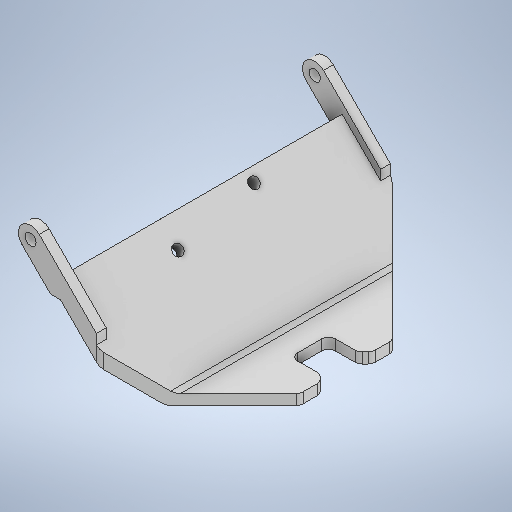
# Autodesk Inventor part: FrontLock
Saved by Autodesk Inventor 2025.1 (Build 291241000, 241)
## iProperties
Created: 2026-05-10
Part Number: FrontLock
Material: Generic
Document SubType Name: Modeling
Designer: User
Density: 1 g/cm^3
Appearance: Default
Author: User
## iProperties of the stored document FrontLock_3DPrint.ipt
Created: 2026-05-12
Part Number: FrontLock_3DPrint
Material: Generic
Document SubType Name: Modeling
Designer: User
Density: 1 g/cm^3
Appearance: Default
Author: User
Autodesk Inventor part; units mm, degrees
ref_plane "YZ Plane" through (0, 0, 0) normal (1, 0, 0) x (0, 1, 0)
sketch "Sketch1" plane through (0, 0, 0) normal (0, 0, 1) x (1, 0, 0)
  circle A0 centre (-6.485281, 1.485281) radius 1.5
  circle A1 centre (-6.485281, 1.485281) radius 1.6
  line L0 (4, 5) -> (-10, 5)
  line L1 (-10, 5) -> (-10, -7)
  line L2 (-3, 0) -> (-5, -2)
  circle A2 centre (-6.485281, 1.485281) radius 3.514719
  line L3 (54.104764, -60.437628) -> (54.104764, 0)
  line L4 (-6.485281, 1.485281) -> (54.104764, -59.104764)
  line L5 (-6.485281, 1.485281) -> (79.201983, 1.485281) construction
  line L6 (-10, -7) -> (-5, -7)
  line L7 (-5, -2) -> (-3, 0)
  line L8 (-5, -2) -> (-3, 0)
  line L9 (-5, -7.5) -> (-10.5, -7.5)
  line L10 (-10.5, -7.5) -> (-10.5, 5.5)
  line L11 (-10.5, 5.5) -> (4, 5.5)
  line L12 (-2.646447, -0.353553) -> (-4.646447, -2.353553)
  circle A3 centre (-6.485281, 1.485281) radius 9.107214
  circle A4 centre (-6.485281, 1.485281) radius 9.841405
  line L13 (0.473643, -5.473643) -> (-0.587018, -6.534303)
  line L14 (0.473643, -5.473643) -> (1.973643, -5.473643) construction
  line L15 (-0.587018, -6.534303) -> (1.534303, -4.412982)
  line L16 (23.809741, -28.809741) -> (24.870402, -27.749081)
  line L17 (1.534303, -4.412982) -> (-0.587018, -6.534303)
  line L18 (-0.587018, -6.534303) -> (22.749081, -29.870402)
  line L19 (22.749081, -29.870402) -> (24.870402, -27.749081)
  line L20 (24.870402, -27.749081) -> (1.534303, -4.412982)
  line L21 (-0.587018, -6.534303) -> (1.534303, -4.412982)
  line L22 (1.534303, -4.412982) -> (-3.826704, 0.948024)
  line L23 (-3.826704, 0.948024) -> (-5.948024, -1.173296)
  line L24 (-5.948024, -1.173296) -> (-0.587018, -6.534303)
  line L25 (22.749081, -29.870402) -> (54.104764, -29.870402)
  line L26 (54.104764, -29.870402) -> (54.104764, -26.870402)
  line L27 (54.104764, -26.870402) -> (22.749081, -26.870402)
  line L28 (22.749081, -26.870402) -> (22.749081, -29.870402)
  point P0 (0, 0)
  point P1 (-3.17704, 0.29836)
  point P2 (-5.29836, -1.822961)
  point P3 (23.991722, -26.870402)
extrude "Extrusion1" add sketch "Sketch1" along normal blind 3 contours A2 L22 L23 L24 | L22 L15 A4 | A4 L4 A3 L22 | A3 L4 A2 L22 | A4 L24 A3 L4 | L15 L20 L27 L28 L4 | L13 L24 A4 | L4 L28 L18 L13 | A2 L4 L23 L22 | L24 L23 L4 A2 | A2 L4 A3 L24 | L28 L27 L20 L16 L4 | L4 L19 L28 | L27 L3 L25 L4 L16 L20 | L4 L25 L19
sketch "Sketch2" plane through (0, 0, 0) normal (0, 0, -1) x (-1, 0, 0)
  line L0 (10, -7) -> (5, -7)
  line L1 (5.29836, -1.822961) -> (-22.749081, -29.870402)
  arc A0 (5.29836, -1.822961) -> (3.17704, 0.29836) centre (6.485281, 1.485281) ccw
  line L2 (-23.991722, -26.870402) -> (3.17704, 0.29836)
  line L3 (-54.104764, -26.870402) -> (-23.991722, -26.870402)
  line L4 (-54.104764, -29.870402) -> (-54.104764, -26.870402)
  line L5 (-22.749081, -29.870402) -> (-54.104764, -29.870402)
  circle A1 centre (6.485281, 1.485281) radius 1.6
  circle A2 centre (6.485281, 1.485281) radius 9.184402
  circle A3 centre (6.485281, 1.485281) radius 9.684402
  point P0 (0, 0)
  point P1 (-1.340645, -4.219325)
  point P2 (0.780675, -6.340645)
  dimension "d11" = 0.5
  constraints: 1 centre point, 1 coincident, 3 other
extrude "Extrusion2" cut sketch "Sketch2" against normal blind 0.2 contours L1 A2 L2 A0 | L1 A3 L2 A2 picked at (2.707023, -2.056333) picked at (0.758356, -5.892503)
sketch "Sketch3" plane through (0, 0, 0) normal (0, 0, -1) x (-1, 0, 0)
  arc A0 (-1.340645, -4.219325) -> (0.780675, -6.340645) centre (6.485281, 1.485281) ccw
  line L0 (-23.991722, -26.870402) -> (-1.340645, -4.219325)
  line L1 (-54.104764, -26.870402) -> (-23.991722, -26.870402)
  line L2 (-54.104764, -29.870402) -> (-54.104764, -26.870402)
  line L3 (-22.749081, -29.870402) -> (-54.104764, -29.870402)
  line L4 (0.780675, -6.340645) -> (-22.749081, -29.870402)
  point P0 (0, 0)
ref_plane "Work Plane1" through (-10, -7, -78.180224) normal (0, 0, -1) x (0, 1, 0)
extrude "Extrusion3" add sketch "Sketch3" along normal up to surface (78.180224 mm away)
sketch "Sketch4" plane through (54.104764, -29.870402, -78.180224) normal (0, 0, -1) x (-1, 0, 0)
  line L0 (30.113042, 3) -> (52.764119, 25.651077)
  line L1 (0, 3) -> (30.113042, 3)
  line L2 (0, 0) -> (0, 3)
  line L3 (31.355683, 0) -> (0, 0)
  line L4 (54.88544, 23.529757) -> (31.355683, 0)
  arc A0 (52.764119, 25.651077) -> (54.88544, 23.529757) centre (60.590046, 31.355683) ccw
  point P0 (54.104764, 29.870402)
extrude "Extrusion4" add sketch "Sketch4" along normal blind 0.2
sketch "Sketch6" plane through (54.104764, -29.870402, -78.380224) normal (0, 0, -1) x (-1, 0, 0)
  line L0 (59.403124, 28.047441) -> (31.355683, 0)
  line L1 (31.355683, 0) -> (0, 0)
  line L2 (0, 0) -> (0, 3)
  line L3 (0, 3) -> (30.113042, 3)
  line L4 (30.113042, 3) -> (57.281804, 30.168762)
  arc A0 (59.403124, 28.047441) -> (57.281804, 30.168762) centre (60.590046, 31.355683) ccw
  circle A1 centre (60.590046, 31.355683) radius 1.6
  point P0 (54.104764, 29.870402)
extrude "Extrusion5" add sketch "Sketch6" along normal blind 2.8
sketch "Sketch7" plane through (22.749081, -29.870402, 3) normal (0, -1, 0) x (1, 0, 0)
  line L0 (9.199091, -15.919764) -> (19.199091, -25.919764)
  line L1 (-21.577508, 14.856835) -> (9.199091, -15.919764)
  line L2 (19.199091, -57.937302) -> (9.199091, -67.937302)
  line L3 (-21.577508, -98.713901) -> (9.199091, -67.937302)
  line L4 (0, -84.180224) -> (-28.047441, -84.180224)
  line L5 (31.355683, -84.180224) -> (0, -84.180224)
  line L6 (31.355683, -84.180224) -> (31.355683, 0)
  line L7 (0, 0) -> (31.355683, 0)
  line L8 (-28.047441, 0) -> (0, 0)
  line L9 (19.199091, -25.919764) -> (29.768225, -36.488898)
  line L10 (19.199091, -57.937302) -> (29.743916, -47.392477)
  line L11 (19.199091, -25.919764) -> (19.199091, -57.937302)
  line L12 (19.199091, -25.919764) -> (51.216629, -25.919764) construction
  line L13 (29.768225, -36.488898) -> (29.743916, -47.392477)
  line L14 (29.743916, -47.392477) -> (8.743968, -47.345658)
  line L15 (8.743968, -47.345658) -> (8.768277, -36.442079)
  line L16 (8.768277, -36.442079) -> (29.768225, -36.488898)
  line L17 (-22.991722, 13.442621) -> (7.784877, -17.333978)
  line L18 (7.784877, -17.333978) -> (17.784877, -27.333978)
  line L19 (17.784877, -27.333978) -> (28.354011, -37.903112)
  line L20 (-22.991722, -97.299688) -> (7.784877, -66.523088)
  line L21 (7.784877, -66.523088) -> (17.784877, -56.523088)
  line L22 (17.784877, -56.523088) -> (28.329702, -45.978263)
  point P0 (-22.749081, -3)
  point P1 (-9.549101, 0)
  point P2 (19.199091, -28.748191)
  point P3 (19.199091, -36.465335)
  point P4 (19.199091, -47.368967)
  point P5 (19.199091, -55.108875)
  point P6 (-9.872259, -84.180224)
  dimension "d20" = 90
  dimension "d21" = 21
  dimension "d22" = 2
  dimension "d23" = 2
  constraints: 24 end point, 2 parallel, 2 perpendicular, 1 horizontal, 1 point on line, 4 other
  measures "d20" angle of L11 L12
  measures "d21" distance of L10.end L14.end
  measures "d22" distance between parallel lines of L1 L17
  measures "d23" distance between parallel lines of L3 L20
extrude "Extrusion6" cut sketch "Sketch7" against normal blind 21
chamfer "Chamfer1" distance 2 angle 45 2 edges at (41.9482, -28.3704, -33.4653) (41.9482, -28.3704, -44.369)
fillet "Fillet1" radius 2 12 edges at (31.5174, -28.3704, -33.4421) (39.9482, -28.3704, -33.4609) (41.9482, -28.3704, -31.4653) (31.493, -28.3704, -44.3457) (39.9482, -28.3704, -44.3645) (41.9482, -28.3704, -46.369) (41.9482, -28.3704, -52.1089) (41.9482, -28.3704, -25.7482) (13.2, -18.2, 3) (12.8768, -17.8768, -81.1802) (22.7491, -29.8704, -38.9285) (23.9917, -26.8704, -38.9285)
sketch "Sketch8" plane through (0, 0, 3) normal (0, 0, 1) x (1, 0, 0)
  arc A0 (-3.17704, 0.29836) -> (-5.29836, -1.822961) centre (-6.485281, 1.485281) ccw
  line L0 (-5.29836, -1.822961) -> (12.371554, -19.492874)
  arc A1 (-0.780675, -6.340645) -> (1.340645, -4.219325) centre (-6.485281, 1.485281) ccw
  line L1 (3.678701, -13.649264) -> (-13.033867, 3.063304)
  line L2 (-0.780675, -6.340645) -> (-2.205297, -7.765266)
  line L3 (-0.780675, -6.340645) -> (1.234043, -6.340645) construction
  line L4 (-0.780675, -6.340645) -> (-5.29836, -1.822961)
  line L5 (-0.780675, -6.340645) -> (-2.205297, -7.765266)
  line L6 (-2.205297, -7.765266) -> (-0.780477, -9.190086)
  line L7 (-0.780477, -9.190086) -> (0.644145, -7.765465)
  line L8 (0.644145, -7.765465) -> (-0.780675, -6.340645)
  point P0 (0, 0)
  dimension "d30" = 135
  dimension "d31" = 2.015
  constraints: 14 end point, 3 parallel, 1 equal length, 1 horizontal, 1 perpendicular, 1 point on line, 1 tangent
  measures "d30" angle of L2 L3
  measures "d31" distance of L6.end L2.end
extrude "Extrusion7" add sketch "Sketch8" against normal up to surface (84.180224 mm away) contours L2 L0 L7 L1
sketch "Sketch9" plane through (0, 0, 3) normal (0, 0, 1) x (1, 0, 0)
  line L0 (-5.29836, -1.822961) -> (-0.780675, -6.340645)
  line L1 (-0.780675, -6.340645) -> (-2.205297, -7.765266)
  arc A0 (-3.17704, 0.29836) -> (-5.29836, -1.822961) centre (-6.485281, 1.485281) ccw
  line L2 (-2.205297, -7.765266) -> (-8.970563, -1)
  point P0 (0, 0)
  constraints: 2 end point, 1 point on circle, 1 tangent
extrude "Extrusion8" add sketch "Sketch9" against normal up to surface (2.8 mm away)
sketch "Sketch10" plane through (54.104764, -29.870402, -81.180224) normal (0, 0, -1) x (-1, 0, 0)
  line L0 (54.88544, 23.529757) -> (56.310061, 22.105136)
  line L1 (54.88544, 23.529757) -> (59.403124, 28.047441)
  arc A0 (59.403124, 28.047441) -> (57.281804, 30.168762) centre (60.590046, 31.355683) ccw
  line L2 (63.075327, 28.870402) -> (56.310061, 22.105136)
  point P0 (54.104764, 29.870402)
extrude "Extrusion9" add sketch "Sketch10" against normal up to surface (2.8 mm away)
sketch "Sketch11" plane through (22.163295, -29.284615, -5.963314) normal (-0.7071068, -0.7071068, 0) x (-0.7071068, 0.7071068, 0)
  line L0 (30.432674, -8.963314) -> (30.432674, 75.21691)
  line L1 (32.447674, -6.163314) -> (32.447674, 72.41691)
  line L2 (32.447674, 72.41691) -> (32.447674, -6.163314)
  line L3 (30.432674, 49.507317) -> (32.447674, 49.507317)
  line L4 (32.447674, 49.507317) -> (32.447674, 58.507317)
  line L5 (32.447674, 58.507317) -> (30.432674, 58.507317)
  line L6 (30.432674, 58.507317) -> (30.432674, 49.507317)
  point P0 (36.379166, -5.963314)
  point P1 (30.432674, 58.507317)
  dimension "d38" = 9
  constraints: 8 end point, 2 parallel, 2 point on line, 1 horizontal, 1 perpendicular
  measures "d38" distance of L4.end L3.end
extrude "Extrusion10" cut sketch "Sketch11" along normal blind 10
sketch "Sketch13" plane through (22.163295, -29.284615, -5.963314) normal (-0.7071068, -0.7071068, 0) x (-0.7071068, 0.7071068, 0)
  line L0 (25.732674, 40.725507) -> (25.732674, 49.207317)
  line L1 (26.232674, 49.707317) -> (25.732674, 49.207317)
  line L2 (26.232674, 49.707317) -> (35.631857, 49.707317)
  line L3 (29.732674, 40.225507) -> (26.232674, 40.225507)
  line L4 (25.732674, 40.725507) -> (26.232674, 40.225507)
  line L5 (30.432674, -8.963314) -> (30.432674, 49.507317)
  line L6 (30.232674, 20.272002) -> (30.232674, 39.725507)
  line L7 (30.232674, 39.725507) -> (29.732674, 40.225507)
  line L8 (35.631857, 49.207317) -> (26.439781, 49.207317)
  line L9 (26.439781, 49.207317) -> (26.232674, 49.000211)
  line L10 (26.232674, 49.000211) -> (26.232674, 40.932613)
  line L11 (26.232674, 40.932613) -> (26.439781, 40.725507)
  line L12 (26.439781, 40.725507) -> (29.939781, 40.725507)
  line L13 (29.939781, 40.725507) -> (30.732674, 39.932613)
  line L14 (30.732674, 39.932613) -> (30.732674, 20.272002)
  line L15 (26.439781, 40.725507) -> (30.432674, 40.725507)
  point P0 (36.379166, -5.963314)
  point P1 (30.432674, 49.207317)
extrude "Extrusion11" add sketch "Sketch13" along normal up to surface (2.014719 mm away) contours L15 L12 L11 L10 L9 L8 L5
sketch "Sketch14" plane through (-8.970563, -1, 3) normal (-0.7071068, -0.7071068, 0) x (-0.7071068, 0.7071068, 0)
  line L0 (-15.782531, 49.895927) -> (-15.782531, 57.963525)
  line L1 (-9.567531, 2.8) -> (-9.567531, 58.470631)
  line L2 (-15.782531, 53.929726) -> (-9.567531, 53.929726)
  circle A0 centre (-12.675031, 53.929726) radius 1.5
  point P0 (-5.636039, 3)
  dimension "d44" = 3
  constraints: 2 end point, 2 midpoint, 1 centre point, 1 perpendicular, 1 point on line
  measures "d44" diameter of A0
extrude "Extrusion12" cut sketch "Sketch14" against normal blind 10
sketch "Sketch15" plane through (22.163295, -29.284615, -5.963314) normal (-0.7071068, -0.7071068, 0) x (-0.7071068, 0.7071068, 0)
  circle A0 centre (25.232674, 20.272002) radius 1.6
  circle A1 centre (25.232674, 20.272002) radius 1.5
  point P0 (36.379166, -5.963314)
  dimension "d47" = 3
  constraints: 1 centre point, 1 coincident
  measures "d47" diameter of A1
extrude "Extrusion13" cut sketch "Sketch15" against normal blind 10 contours A1
sketch "Sketch16" plane through (0.644145, -7.765465, -55.470631) normal (0, 0, -1) x (-0.7071068, -0.7071068, 0)
  line L0 (0, -4.2) -> (2.5, -4.2)
  line L1 (0, 7.215) -> (0, -4.2)
  line L2 (0, 7.215) -> (0.484183, 7.215)
  line L3 (0.484183, 7.215) -> (2.5, 5.199183)
  line L4 (2.5, -4.2) -> (2.5, 5.199183)
  line L5 (0, 2.015) -> (2.014719, 2.015)
  line L6 (2.5, -4.2) -> (2.5, 5.199183)
  line L7 (2.014719, 0) -> (0, 0)
  line L8 (2.014719, 2.015) -> (2.014719, 0)
  point P0 (-5.035534, 5.946492)
extrude "Extrusion14" cut sketch "Sketch16" against normal up to surface (0.3 mm away) contours L1 L5 L8 L7
chamfer "Chamfer2" distance 1 angle 45 1 edges at (-0.0682, -8.4778, -64.4706)
sketch "Sketch17" plane through (0, 0, 3) normal (0, 0, 1) x (1, 0, 0)
  arc A0 (-3.17704, 0.29836) -> (-8.970563, -1) centre (-6.485281, 1.485281) ccw
  line L0 (12.371554, -15.250233) -> (-3.17704, 0.29836)
  line L1 (12.371554, -15.250233) -> (12.371554, -19.492874)
  line L2 (12.371554, -19.492874) -> (12.371554, -1.590045)
  line L3 (16.660681, -16.690119) -> (-8.999554, 8.970117)
  point P0 (0, 0)
  point P1 (12.371554, -12.400991)
  point P2 (-4, 3.970563)
  constraints: 4 end point, 1 parallel, 1 point on line, 1 tangent
extrude "Extrusion15" add sketch "Sketch17" against normal up to surface (2.8 mm away)
sketch "Sketch18" plane through (54.104764, -29.870402, -81.180224) normal (0, 0, -1) x (-1, 0, 0)
  line L0 (57.281804, 30.168762) -> (42.056369, 14.943327)
  line L1 (41.733211, 17.469411) -> (58.104764, 33.840964)
  line L2 (40.642156, 13.529113) -> (42.056369, 14.943327)
  line L3 (41.733211, 14.620168) -> (41.733211, 17.469411)
  arc A0 (63.075327, 28.870402) -> (57.281804, 30.168762) centre (60.590046, 31.355683) ccw
  point P0 (54.104764, 29.870402)
extrude "Extrusion16" add sketch "Sketch18" against normal up to surface (2.8 mm away)
sketch "Sketch19" plane through (0, 0, 3) normal (0, 0, 1) x (1, 0, 0)
  line L0 (-0.780477, -9.190086) -> (0.644145, -7.765465)
  line L1 (0.644145, -7.765465) -> (12.371554, -19.492874)
  line L2 (0.644145, -7.765465) -> (2.068965, -9.190285)
  line L3 (0.644145, -7.765465) -> (2.659145, -7.765465) construction
  line L4 (2.068965, -9.190285) -> (-0.780477, -9.190086)
  point P0 (0, 0)
  dimension "d59" = 2.015
  dimension "d60" = 45
  constraints: 6 end point, 1 equal length, 1 horizontal, 1 point on line
  measures "d59" distance of L0.end L2.end
  measures "d60" angle of L2 L3
ref_plane "Work Plane2" through (-5.37687, -31.24141, -20.735316) normal (0, 0, 1) x (0.7071068, 0.7071068, 0)
extrude "Extrusion17" add sketch "Sketch19" against normal up to surface (23.735316 mm away)
equation "\"d24\" = d21"
equation "\"d32\" = d21"
body "Solid1"
